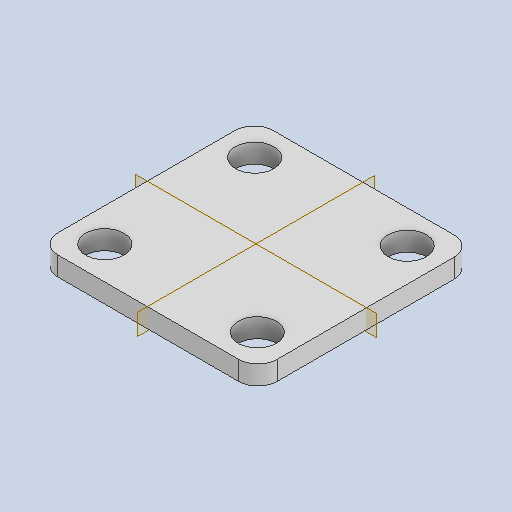
# Autodesk Inventor part: энкодер
Saved by Autodesk Inventor 2024.2 (Build 282272000, 272)
## iProperties
Created: 2025-11-27
Part Number: энкодер
Material: Типовые
Document SubType Name: Modeling
Designer: katya_notebook
Density: 1 g/cm^3
Appearance: По умолчанию
Author: katya_notebook
Autodesk Inventor part; units mm, degrees
ref_plane "XZ Plane" through (0, 0, 0) normal (0, 1, 0) x (-1, 0, 0)
sketch "Эскиз1" plane through (0, 0, 0) normal (0, 1, 0) x (-1, 0, 0)
  line L0 (-11.45, -11.25) -> (11.45, -11.25)
  line L1 (11.45, -11.25) -> (11.45, 11.25)
  line L2 (11.45, 11.25) -> (-11.45, 11.25)
  line L3 (-11.45, 11.25) -> (-11.45, -11.25)
  line L4 (-11.45, -11.25) -> (11.45, 11.25) construction
  line L5 (11.45, -11.25) -> (-11.45, 11.25) construction
  point P0 (0, 0)
  dimension "d0" = 22.5
  dimension "d1" = 22.9
  constraints: 12 end point, 2 midpoint, 2 parallel, 1 horizontal, 1 perpendicular
  measures "d0" distance of L0.end L1.end
  measures "d1" distance of L1.end L2.end
extrude "Выдавливание1" add sketch "Эскиз1" along normal blind 2
sketch "Эскиз2" plane through (0, 2, 0) normal (0, 1, 0) x (1, 0, 0)
  line L0 (-11.45, 11.25) -> (-11.45, -11.25) projected
  line L1 (-11.45, -11.25) -> (0, 0)
  circle A0 centre (-7.9663, -7.8272) radius 2
  line L2 (15.4928, 0) -> (-16.8416, 0)
  line L3 (0, -16.9938) -> (0, 16.458)
  circle A1 centre (-7.9663, 7.8272) radius 2
  circle A2 centre (7.9663, -7.8272) radius 2
  circle A3 centre (7.9663, 7.8272) radius 2
  dimension "d8" = 4
  constraints: 6 end point, 4 centre point, 3 symmetric about line, 1 horizontal, 1 point on line, 1 vertical, 3 other
  measures "d8" diameter of A0
extrude "Выдавливание2" cut sketch "Эскиз2" against normal blind 2 contours A0 L1 | L1 A0 | A1 | A2 | A3
fillet "Сопряжение1" radius 2 4 edges at (-11.45, 1, 11.25) (11.45, 1, 11.25) (11.45, 1, -11.25) (-11.45, 1, -11.25)
